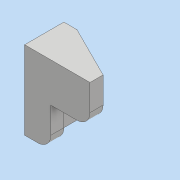
# Autodesk Inventor part: 5
Saved by Autodesk Inventor 2017 (Build 210142000, 142)
## iProperties
Part Number: 5
Material: 一般
Document SubType Name: Modeling
Designer: d8910
Density: 1 g/cm^3
Appearance: 預設
Author: d8910
Autodesk Inventor part; units mm, degrees
ref_plane "YZ Plane" through (0, 0, 0) normal (1, 0, 0) x (0, 1, 0)
ref_plane "XZ Plane" through (0, 0, 0) normal (0, 1, 0) x (-1, 0, 0)
ref_plane "XY Plane" through (0, 0, 0) normal (0, 0, 1) x (1, 0, 0)
sketch "草圖1" plane through (0, 0, 0) normal (0, 1, 0) x (-1, 0, 0)
  line L0 (10, 15) -> (-15, 15)
  line L1 (-15, 15) -> (-15, 5)
  line L2 (-10, 0) -> (0, 0)
  line L3 (10, 0) -> (10, 15)
  line L4 (10, 15) -> (0, 15)
  line L5 (0, 0) -> (0, -10)
  line L6 (5, -15) -> (10, -15)
  line L7 (10, -15) -> (10, 15)
  arc A0 (0, -10) -> (5, -15) centre (5, -10) ccw
  arc A1 (-15, 5) -> (-10, 0) centre (-10, 5) ccw
  point P0 (-15, 0)
  point P1 (0, -15)
  dimension "d0" = 15
  dimension "d1" = 10
  dimension "d2" = 30
  dimension "d3" = 25
  dimension "d4" = 5
  constraints: 16 end point, 4 parallel, 4 point on circle, 4 point on line, 4 tangent, 2 centre point, 2 coincident, 2 horizontal, 2 perpendicular, 1 equal radius
  measures "d0" distance of L0.end point (-15, 0)
  measures "d1" distance of point (0, -15) L6.end
  measures "d2" distance of L6.end L0.start
  measures "d3" distance of L0.start L0.end
  measures "d4" radius of A0
extrude "擠出1" add sketch "草圖1" along normal blind 5
sketch "草圖2" plane through (-10, 0, -15) normal (-1, 0, 0) x (0, 0, 1)
  line L0 (30, 0) -> (20, 0) construction
  line L1 (20, 0) -> (20, 5) construction
  line L2 (30, 5) -> (20, 5) construction
  line L3 (30, 0) -> (30, 5) construction
  line L4 (20, 0) -> (15, 0) construction
  line L5 (15, 0) -> (15, 5) construction
  line L6 (20, 5) -> (15, 5) construction
  line L7 (20, 0) -> (20, 5) construction
  line L8 (15, 0) -> (5, 0) construction
  line L9 (5, 0) -> (5, 5) construction
  line L10 (15, 5) -> (5, 5) construction
  line L11 (15, 0) -> (15, 5) construction
  line L12 (5, 0) -> (0, 0) construction
  line L13 (0, 0) -> (0, 5) construction
  line L14 (5, 5) -> (0, 5) construction
  line L15 (5, 0) -> (5, 5) construction
  line L16 (30, 0) -> (30, 5) projected
  line L17 (30, 5) -> (20, 5)
  line L18 (20, 10) -> (20, 15)
  line L19 (20, 15) -> (30, 15)
  line L20 (30, 15) -> (30, 5)
  line L21 (15, 5) -> (5, 5) projected
  line L22 (20, 10) -> (5, 10)
  line L23 (5, 5) -> (20, 5)
  line L24 (0, 5) -> (30, 5) projected
  line L25 (0, 5) -> (5, 5)
  line L26 (5, 10) -> (5, 25)
  line L27 (5, 25) -> (5, 25)
  line L28 (0, 20) -> (0, 5)
  arc A0 (5, 25) -> (0, 20) centre (5, 20) ccw
  point P0 (0, 25)
  dimension "d7" = 5
  dimension "d8" = 10
  dimension "d9" = 10
  dimension "d10" = 5
  dimension "d11" = 20
  dimension "d12" = 5
  constraints: 20 end point, 5 parallel, 3 horizontal, 2 perpendicular, 2 point on circle, 2 point on line, 2 tangent, 1 centre point
  measures "d7" distance of L26.end point (0, 25)
  measures "d8" distance of L18.end L19.end
  measures "d9" distance between parallel lines of L2 L19
  measures "d10" distance between parallel lines of L10 L22
  measures "d11" distance of point (0, 25) L13.end
  measures "d12" radius of A0
extrude "擠出2" add sketch "草圖2" against normal blind 5
sketch "草圖3" plane through (-10, 0, 15) normal (0, 0, 1) x (1, 0, 0)
  line L0 (0, 0) -> (25, 0) construction
  line L1 (25, 0) -> (25, 5) construction
  line L2 (5, 5) -> (25, 5) construction
  line L3 (5, 15) -> (5, 5) construction
  line L4 (0, 15) -> (5, 15) construction
  line L5 (0, 0) -> (0, 15) construction
  line L6 (5, 5) -> (25, 5) projected
  line L7 (5, 15) -> (25, 5)
  line L8 (25, 5) -> (5, 5)
  line L9 (5, 5) -> (5, 15)
  point P0 (10, 0)
  constraints: 6 end point, 1 collinear, 1 perpendicular
extrude "擠出3" add sketch "草圖3" against normal blind 5
